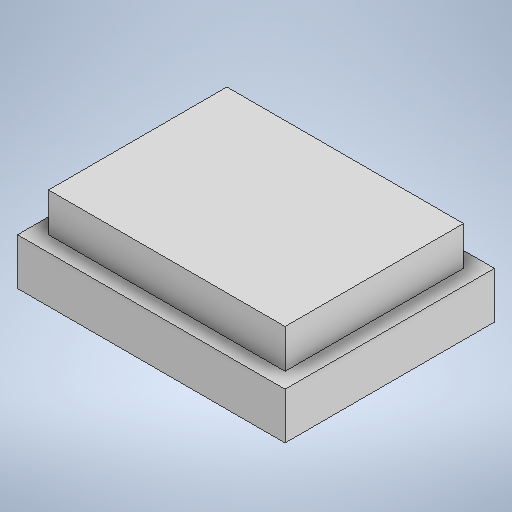
# Autodesk Inventor part: Arduino_Shield_ph
Saved by Autodesk Inventor 2025 (Build 290162000, 162)
## iProperties
Created: 2026-07-08
Part Number: Arduino_Shield_ph
Material: Generisch
Document SubType Name: Modeling
Designer: wavid
Density: 1 g/cm^3
Appearance: Vorgabe
Author: wavid
Autodesk Inventor part; units mm, degrees
ref_plane "YZ Plane" through (0, 0, 0) normal (1, 0, 0) x (0, 1, 0)
ref_plane "XZ Plane" through (0, 0, 0) normal (0, 1, 0) x (-1, 0, 0)
sketch "Skizze1" plane through (0, 0, 0) normal (0, 0, 1) x (1, 0, 0)
  line L0 (0, 0) -> (69, 0)
  line L1 (69, 0) -> (69, 54)
  line L2 (69, 54) -> (0, 54)
  line L3 (0, 54) -> (0, 0)
  constraints: 8 end point, 2 parallel, 1 horizontal, 1 perpendicular
extrude "Extrusion1" add sketch "Skizze1" along normal blind 12
ref_plane "Arbeitsebene1" through (0, 0, 12) normal (0, 0, 1) x (1, 0, 0)
sketch "Skizze2" plane through (0, 0, 12) normal (0, 0, 1) x (1, 0, 0)
  line L0 (4, 4) -> (65, 4)
  line L1 (65, 4) -> (65, 50)
  line L2 (65, 50) -> (4, 50)
  line L3 (4, 50) -> (4, 4)
  constraints: 8 end point, 2 parallel, 1 horizontal, 1 perpendicular
extrude "Extrusion2" add sketch "Skizze2" along normal blind 10 separate body
